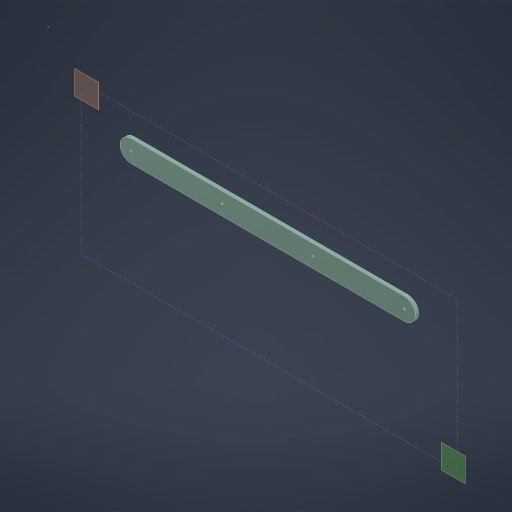
# Autodesk Inventor part: foot4
Saved by Autodesk Inventor 2024.2 (Build 282272000, 272)
## iProperties
Created: 2024-06-20
Part Number: foot4
Material: Generic
Document SubType Name: Modeling
Designer: Moe
Density: 1 g/cm^3
Appearance: Default
Author: Moe
Autodesk Inventor part; units mm, degrees
ref_plane "YZ Plane" through (0, 0, 0) normal (1, 0, 0) x (0, 1, 0)
ref_plane "XZ Plane" through (0, 0, 0) normal (0, 1, 0) x (-1, 0, 0)
ref_plane "XY Plane" through (0, 0, 0) normal (0, 0, 1) x (1, 0, 0)
ref_plane "Work Plane2" through (35.545, -31.609, 1.6) normal (0, 0, 1) x (1, 0, 0)
sketch "Sketch2" plane through (35.545, -31.609, 1.6) normal (0, 0, 1) x (1, 0, 0)
  line L0 (-4.7778, 3.1171) -> (341.5466, 3.1925) construction
  line L1 (341.5466, 3.1925) -> (341.5765, -133.848) construction
  line L2 (341.5765, -133.848) -> (-4.7479, -133.9235) construction
  line L3 (-4.7479, -133.9235) -> (-4.7778, 3.1171) construction
  point P0 (-35.545, 31.609)
  constraints: 2 other
ref_plane "Work Plane1" through (371.545, -162.609, 0) normal (0, 0, -1) x (-1, 0, 0)
sketch "Sketch9" plane through (371.545, -162.609, 0) normal (0, 0, -1) x (-1, 0, 0)
  line L0 (336, 131) -> (0, 131) projected
  line L1 (-2, 129) -> (-2, 2) projected
  line L2 (-1.9796, 129.2846) -> (-2, 129) projected
  line L3 (-1.919, 129.5635) -> (-1.9796, 129.2846) projected
  line L4 (-1.8193, 129.8308) -> (-1.919, 129.5635) projected
  line L5 (-1.6825, 130.0813) -> (-1.8193, 129.8308) projected
  line L6 (-1.5115, 130.3097) -> (-1.6825, 130.0813) projected
  line L7 (-1.3097, 130.5115) -> (-1.5115, 130.3097) projected
  line L8 (-1.0813, 130.6825) -> (-1.3097, 130.5115) projected
  line L9 (-0.8308, 130.8193) -> (-1.0813, 130.6825) projected
  line L10 (-0.5635, 130.919) -> (-0.8308, 130.8193) projected
  line L11 (-0.2846, 130.9796) -> (-0.5635, 130.919) projected
  line L12 (0, 131) -> (-0.2846, 130.9796) projected
  circle A0 centre (2.362, 128.645) radius 1.1 projected
  circle A1 centre (68.695, 128.645) radius 1.1 projected
  circle A2 centre (135.028, 128.645) radius 1.1 projected
  circle A3 centre (201.361, 128.645) radius 1.1 projected
  circle A4 centre (267.694, 128.645) radius 1.1 projected
  circle A5 centre (334.027, 128.645) radius 1.1 projected
  line L13 (338, 2) -> (338, 129) projected
  line L14 (338, 129) -> (337.9796, 129.2846) projected
  line L15 (337.9796, 129.2846) -> (337.919, 129.5635) projected
  line L16 (337.919, 129.5635) -> (337.8193, 129.8308) projected
  line L17 (337.8193, 129.8308) -> (337.6825, 130.0813) projected
  line L18 (337.6825, 130.0813) -> (337.5115, 130.3097) projected
  line L19 (337.5115, 130.3097) -> (337.3097, 130.5115) projected
  line L20 (337.3097, 130.5115) -> (337.0813, 130.6825) projected
  line L21 (337.0813, 130.6825) -> (336.8308, 130.8193) projected
  line L22 (336.8308, 130.8193) -> (336.5635, 130.919) projected
  line L23 (336.5635, 130.919) -> (336.2846, 130.9796) projected
  line L24 (336.2846, 130.9796) -> (336, 131) projected
  line L25 (0, 0) -> (336, 0) projected
  line L26 (336, 0) -> (336.2846, 0.0204) projected
  line L27 (336.2846, 0.0204) -> (336.5635, 0.081) projected
  line L28 (336.5635, 0.081) -> (336.8308, 0.1807) projected
  line L29 (336.8308, 0.1807) -> (337.0813, 0.3175) projected
  line L30 (337.0813, 0.3175) -> (337.3097, 0.4885) projected
  line L31 (337.3097, 0.4885) -> (337.5115, 0.6903) projected
  line L32 (337.5115, 0.6903) -> (337.6825, 0.9187) projected
  line L33 (337.6825, 0.9187) -> (337.8193, 1.1692) projected
  line L34 (337.8193, 1.1692) -> (337.919, 1.4365) projected
  line L35 (337.919, 1.4365) -> (337.9796, 1.7154) projected
  line L36 (337.9796, 1.7154) -> (338, 2) projected
  circle A6 centre (334.02, 2.37) radius 1.1 projected
  circle A7 centre (267.687, 2.37) radius 1.1 projected
  circle A8 centre (201.354, 2.37) radius 1.1 projected
  circle A9 centre (135.021, 2.37) radius 1.1 projected
  circle A10 centre (68.688, 2.37) radius 1.1 projected
  circle A11 centre (2.355, 2.37) radius 1.1 projected
  line L37 (-0.2846, 0.0204) -> (0, 0) projected
  line L38 (-0.5635, 0.081) -> (-0.2846, 0.0204) projected
  line L39 (-0.8308, 0.1807) -> (-0.5635, 0.081) projected
  line L40 (-1.0813, 0.3175) -> (-0.8308, 0.1807) projected
  line L41 (-1.3097, 0.4885) -> (-1.0813, 0.3175) projected
  line L42 (-1.5115, 0.6903) -> (-1.3097, 0.4885) projected
  line L43 (-1.6825, 0.9187) -> (-1.5115, 0.6903) projected
  line L44 (-1.8193, 1.1692) -> (-1.6825, 0.9187) projected
  line L45 (-1.919, 1.4365) -> (-1.8193, 1.1692) projected
  line L46 (-1.9796, 1.7154) -> (-1.919, 1.4365) projected
  line L47 (-2, 2) -> (-1.9796, 1.7154) projected
  circle A12 centre (41.979, 103.44) radius 1.1 projected
  circle A13 centre (125.979, 103.44) radius 1.1 projected
  circle A14 centre (210.039, 103.527) radius 1.1 projected
  circle A15 centre (294.039, 103.527) radius 1.1 projected
  point P0 (371.545, 162.609)
ref_plane "Work Plane3" through (371.545, -162.609, 0) normal (0, 0, 1) x (1, 0, 0)
sketch "Sketch10" plane through (371.545, -162.609, 0) normal (0, 0, 1) x (1, 0, 0)
  circle A0 centre (-294.039, 103.527) radius 1.1 projected
  circle A1 centre (-210.039, 103.527) radius 1.1 projected
  circle A2 centre (-125.979, 103.44) radius 1.1 projected
  circle A3 centre (-41.979, 103.44) radius 1.1 projected
  line L0 (-294.039, 113.527) -> (-41.979, 113.527)
  line L1 (-31.979, 103.527) -> (-31.979, 103.527)
  line L2 (-41.979, 93.527) -> (-294.039, 93.527)
  line L3 (-304.039, 103.527) -> (-304.039, 103.527)
  arc A4 (-31.979, 103.527) -> (-41.979, 113.527) centre (-41.979, 103.527) ccw
  arc A5 (-41.979, 93.527) -> (-31.979, 103.527) centre (-41.979, 103.527) ccw
  arc A6 (-294.039, 113.527) -> (-304.039, 103.527) centre (-294.039, 103.527) ccw
  arc A7 (-304.039, 103.527) -> (-294.039, 93.527) centre (-294.039, 103.527) ccw
  point P0 (-371.545, 162.609)
  point P1 (-31.979, 103.527)
  dimension "d89" = 10
  dimension "d90" = 10
  dimension "d91" = 10
  dimension "d92" = 10
  dimension "d93" = 10
  constraints: 8 end point, 8 point on circle, 8 tangent, 4 centre point, 3 equal radius, 2 parallel, 1 horizontal, 1 perpendicular
  measures "d89" distance from line of A0.centre L0
  measures "d90" distance from line of A0.centre L2
  measures "d91" distance from line of L3 A0.centre
  measures "d92" distance from line of L1 A3.centre
  measures "d93" radius of A4
extrude "Extrusion4" add sketch "Sketch10" along normal blind 3
body "Solid1"
